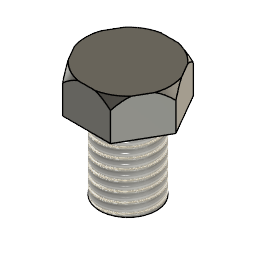
Set Screw (Autodesk Fusion 360 design; units mm, degrees)
Autodesk Fusion 360 part; units mm, degrees
sketch "Sketch1" plane through (0, 0, 0) normal (0, 0, 1) x (1, 0, 0)
  circle A0 centre (0, 0) radius 4.7625
  dimension "d1" = 9.525
  constraint coincident A0.centre origin
  measures "d1" diameter of A0
extrude "Extrude1" add sketch "Sketch1" along normal blind 12.7
thread "Thread1" "ANSI Unified Screw Threads 0.375 3/8-16 UNC 3/8-16 UNC 3A" major diameter 9.4056 minor diameter 7.6327 pitch 1.5875 angle 60 resizes the face on face at (4.7388, -0.4742, 8.4667)
sketch "Sketch2" plane through (0, 0, 12.7) normal (0, 0, 1) x (-1, 0, 0)
  circle A0 centre (0, 0) radius 4.7028
  circle A1 centre (0, 0) radius 7.9375
  line L0 (-7.9375, 0) -> (-3.9688, -6.8741)
  line L1 (-3.9688, -6.8741) -> (3.9687, -6.8741)
  line L2 (3.9687, -6.8741) -> (7.9375, 0)
  line L3 (7.9375, 0) -> (3.9688, 6.8741)
  line L4 (3.9688, 6.8741) -> (-3.9687, 6.8741)
  line L5 (-3.9687, 6.8741) -> (-7.9375, 0)
  dimension "d6" = 15.875
  constraint coincident A0.centre A1.centre
  constraint coincident A1 L0.start
  measures "d6" diameter of A1
extrude "Extrude2" add sketch "Sketch2" along normal blind 6.35 contours A0 | L0 L1 L2 L3 L4 L5
sketch "Sketch5" plane through (0, 0, 0) normal (0, 1, 0) x (1, 0, 0)
  line L0 (-7.021, -19.05) -> (-7.9375, -17.4625)
  line L1 (-7.9375, -12.7) -> (-7.9375, -19.05)
  line L2 (-7.9375, -19.05) -> (-3.9688, -19.05)
  dimension "d13" = 1.5875
  dimension "d14" = 150
  constraint coincident L0.end L1
  constraint coincident L0.start L2
  measures "d13" distance of L0.end L1.end
  measures "d14" angle of L0 L1
revolve "Revolve1" cut sketch "Sketch5" angle 360 about axis through (0, 0, 0) along (0, 0, -1)
